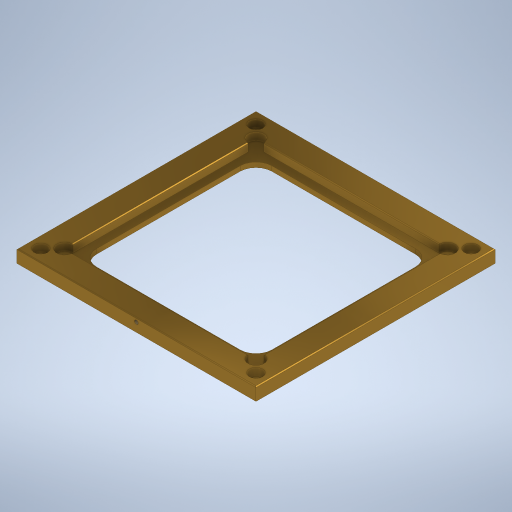
# Autodesk Inventor part: Suporte base da mesa
Saved by Autodesk Inventor 2023 (Build 270158000, 158)
## iProperties
Created: 2023-04-01
Part Number: Suporte base da mesa
Material: Brass, Soft Yellow
Document SubType Name: Sheet Metal
Designer: Mateus PC
Density: 8.47 g/cm^3
Sheet Metal Rule: Default_mm
Appearance: Brass - Satin
Mass: 588.889 g
Surface Area: 302.562 cm^2
Volume: 69.5265 cm^3
Author: Mateus PC
Autodesk Inventor part; units mm, degrees
note: some values were not read from the file. Chosen so that the rebuilt part matches the saved one: direction of "Furo1"; direction of "Furo2".
ref_plane "YZ Plane" through (0, 0, 0) normal (1, 0, 0) x (0, 1, 0)
ref_plane "XZ Plane" through (0, 0, 0) normal (0, 1, 0) x (-1, 0, 0)
ref_plane "XY Plane" through (0, 0, 0) normal (0, 0, 1) x (1, 0, 0)
sketch "Esboço1" plane through (0, 0, 0) normal (0, 1, 0) x (-1, 0, 0)
  line L0 (0, 0) -> (150, 0)
  line L1 (150, 0) -> (150, -150)
  line L2 (150, -150) -> (0, -150)
  line L3 (0, -150) -> (0, 0)
  dimension "d0" = 150
  dimension "d1" = 150
  constraints: 8 end point, 2 parallel, 1 horizontal, 1 perpendicular
  measures "d0" distance of L1.end L2.end
  measures "d1" distance of L0.end L1.end
extrude "Extrusão1" add sketch "Esboço1" along normal blind 8
sketch "Esboço2" plane through (0, 8, 0) normal (0, 1, 0) x (1, 0, 0)
  line L0 (-135, 15) -> (-15, 15)
  line L1 (-15, 15) -> (-15, 135)
  line L2 (-15, 135) -> (-135, 135)
  line L3 (-135, 135) -> (-135, 15)
  line L4 (0, 150) -> (-150, 150) projected
  line L5 (0, 0) -> (0, 150) projected
  point P0 (-75, 135)
  point P1 (-75, 150)
  point P2 (0, 75)
  point P3 (-135, 75)
  dimension "d4" = 120
  dimension "d5" = 120
  dimension "d6" = 0
  dimension "d7" = 0
  constraints: 8 end point, 4 midpoint, 2 parallel, 1 horizontal, 1 perpendicular
  measures "d4" distance of L2.end L0.start
  measures "d5" distance of L1.end L2.end
  measures "d6" horizontal distance of point (-75, 135) point (-75, 150)
  measures "d7" vertical distance of point (0, 75) point (-135, 75)
extrude "Extrusão2" cut sketch "Esboço2" against normal blind 5
sketch "Esboço3" plane through (0, 3, 0) normal (0, 1, 0) x (1, 0, 0)
  line L0 (-120, 20) -> (-30, 20)
  line L1 (-20, 30) -> (-20, 120)
  line L2 (-30, 130) -> (-120, 130)
  line L3 (-130, 120) -> (-130, 30)
  line L4 (-135, 15) -> (-135, 135) projected
  line L5 (-135, 135) -> (-15, 135) projected
  arc A0 (-120, 130) -> (-130, 120) centre (-120, 120) ccw
  arc A1 (-20, 120) -> (-30, 130) centre (-30, 120) ccw
  arc A2 (-30, 20) -> (-20, 30) centre (-30, 30) ccw
  arc A3 (-130, 30) -> (-120, 20) centre (-120, 30) ccw
  point P0 (0, 0)
  point P1 (-130, 20)
  point P2 (-20, 130)
  point P3 (-20, 20)
  point P4 (-130, 130)
  point P5 (-135, 75)
  point P6 (-130, 75)
  point P7 (-75, 135)
  point P8 (-75, 130)
  dimension "d10" = 110
  dimension "d11" = 0
  dimension "d12" = 0
  dimension "d52" = 10
  constraints: 8 end point, 8 point on circle, 8 point on line, 8 tangent, 4 centre point, 4 midpoint, 3 equal radius, 2 parallel, 2 perpendicular, 1 horizontal
  measures "d10" distance of point (-130, 130) point (-130, 20)
  measures "d11" vertical distance of point (-135, 75) point (-130, 75)
  measures "d12" horizontal distance of point (-75, 135) point (-75, 130)
  measures "d52" radius of A0
extrude "Extrusão3" cut sketch "Esboço3" against normal up to surface (3 mm away)
sketch "Esboço4" plane through (0, 8, 0) normal (0, 1, 0) x (1, 0, 0)
  circle A0 centre (-15, 15) radius 5
  circle A1 centre (-135, 15) radius 5
  circle A2 centre (-135, 135) radius 5
  circle A3 centre (-15, 135) radius 5
  line L0 (-15, 135) -> (-15, 15) projected
  line L1 (-15, 15) -> (-135, 15) projected
  line L2 (-135, 15) -> (-135, 135) projected
  line L3 (-135, 135) -> (-15, 135) projected
  point P0 (0, 0)
  dimension "d15" = 10
  dimension "d16" = 0
  dimension "d17" = 0
  dimension "d18" = 0
  dimension "d19" = 0
  dimension "d20" = 0
  dimension "d21" = 0
  dimension "d22" = 0
  dimension "d23" = 0
  constraints: 4 centre point, 3 equal radius
  measures "d15" diameter of A0
  measures "d16" distance from line of A0.centre L0
  measures "d17" distance from line of L1 A0.centre
  measures "d18" distance from line of L1 A1.centre
  measures "d19" distance from line of L2 A1.centre
  measures "d20" distance from line of L2 A2.centre
  measures "d21" distance from line of L3 A2.centre
  measures "d22" distance from line of L3 A3.centre
  measures "d23" distance from line of L0 A3.centre
extrude "Extrusão4" cut sketch "Esboço4" against normal blind 5 contours A0 L1 L0 | L0 L1 A0 | L0 L3 A3 | A3 L3 L0 | L1 L2 A1 | A1 L2 L1 | L3 L2 A2 | A2 L2 L3
sketch "Esboço5" plane through (-150, 0, 0) normal (0, 0, 1) x (1, 0, 0)
  line L0 (130, 3) -> (20, 3) projected
  line L1 (0, 8) -> (150, 8) projected
  point P0 (150, 0)
  point P1 (75, 5.5)
  point P2 (75, 8)
  dimension "d26" = 5
  dimension "d27" = 2.5
  dimension "d28" = 0
  constraints: 1 midpoint
  measures "d26" distance between parallel lines of L1 L0
  measures "d27" distance from line of L1 point (75, 5.5)
  measures "d28" horizontal distance of point (75, 8) point (75, 5.5)
hole "Furo1" at (-75, 5.5, 0) direction (0, 0, -1) diameter 2.459 end up to surface thread size "M3x0.5" class "6H" standard "ISO Metric profile"
sketch "Esboço6" plane through (0, 8, 0) normal (0, 1, 0) x (1, 0, 0)
  line L0 (-150, 150) -> (-150, 0) projected
  line L1 (-135, 20) -> (-135, 130) projected
  line L2 (0, 150) -> (-150, 150) projected
  line L3 (0, 0) -> (0, 150) projected
  line L4 (-150, 0) -> (0, 0) projected
  point P0 (-142.5, 7.5)
  point P1 (-142.5, 142.5)
  point P2 (-7.5, 142.5)
  point P3 (-7.5, 7.5)
  point P4 (-135, 75)
  point P5 (-150, 75)
  dimension "d36" = 7.5
  dimension "d37" = 15
  dimension "d38" = 7.5
  dimension "d39" = 7.5
  dimension "d40" = 7.5
  dimension "d41" = 7.5
  dimension "d42" = 7.5
  dimension "d43" = 7.5
  dimension "d44" = 7.5
  constraints: 2 midpoint
  measures "d36" distance from line of L0 point (-142.5, 142.5)
  measures "d37" distance of point (-135, 75) point (-150, 75)
  measures "d38" distance from line of L2 point (-142.5, 142.5)
  measures "d39" distance from line of L2 point (-7.5, 142.5)
  measures "d40" distance from line of L3 point (-7.5, 142.5)
  measures "d41" distance from line of L3 point (-7.5, 7.5)
  measures "d42" distance from line of L4 point (-7.5, 7.5)
  measures "d43" distance from line of L4 point (-142.5, 7.5)
  measures "d44" distance from line of L0 point (-142.5, 7.5)
hole "Furo2" at (-142.5, 8, -7.5) at (-142.5, 8, -142.5) at (-7.5, 8, -142.5) at (-7.5, 8, -7.5) direction (0, -1, 0) diameter 5 depth 8 counterbore diameter 8.5 counterbore depth 5
chamfer "Chamfer1" distance 0.5 angle 45 8 edges at (-150, 8, -75) (-75, 8, -150) (0, 8, -75) (-75, 8, 0) (-75, 8, -15) (-15, 8, -75) (-75, 8, -135) (-135, 8, -75)
equation "\"d27\" = 0.5 * d26"
equation "\"d36\" = 0.5 * d37"
equation "\"d38\" = d36"
equation "\"d39\" = d36"
equation "\"d40\" = d36"
equation "\"d41\" = d40"
equation "\"d42\" = d41"
equation "\"d43\" = d42"
equation "\"d44\" = d43"
equation "\"Raio_vergadura\" = Espessura"
equation "\"Largura_alívio_de_vergadura\" = Espessura"
equation "\"Profundidade_alívio_de_vergadura\" = 0.5 * Espessura"
equation "\"Tamanho_alívio_de_dobra\" = 4 * Espessura"
equation "\"Remanescente_mínimo\" = 2 * Espessura"
equation "\"Raiodetransição\" = Raio_vergadura"
equation "\"Tamanho_de_raio_de_Jacobi\" = Raio_vergadura"
equation "\"TamanhoFolga\" = Espessura"
equation "\"Espessura\" = 0.5"
